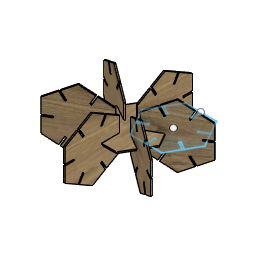
EFDI - MT03 - NDQ (Autodesk Fusion 360 design; units mm, degrees)
Autodesk Fusion 360 part; units mm, degrees
sketch "Boceto1" plane through (0, 0, 0) normal (0, 0, 1) x (1, 0, 0)
  line L0 (50, 110) -> (50, -10)
  line L1 (48.4, -10) -> (48.4, 10)
  line L2 (48.4, 10) -> (51.6, 10)
  line L3 (51.6, 10) -> (51.6, -10)
  line L4 (85.441, 31.3856) -> (102.7615, 21.3856)
  line L5 (101.1615, 18.6144) -> (83.841, 28.6144)
  line L6 (83.841, 28.6144) -> (85.441, 31.3856)
  line L7 (83.841, 71.3856) -> (101.1615, 81.3856)
  line L8 (102.7615, 78.6144) -> (85.441, 68.6144)
  line L9 (85.441, 68.6144) -> (83.841, 71.3856)
  line L10 (48.4, 90) -> (48.4, 110)
  line L11 (51.6, 110) -> (51.6, 90)
  line L12 (51.6, 90) -> (48.4, 90)
  line L13 (14.559, 68.6144) -> (-2.7615, 78.6144)
  line L14 (-1.1615, 81.3856) -> (16.159, 71.3856)
  line L15 (16.159, 71.3856) -> (14.559, 68.6144)
  line L16 (16.159, 28.6144) -> (-1.1615, 18.6144)
  line L17 (-2.7615, 21.3856) -> (14.559, 31.3856)
  line L18 (14.559, 31.3856) -> (16.159, 28.6144)
  line L19 (84.641, -10) -> (101.1615, 18.6144)
  line L20 (102.7615, 21.3856) -> (119.282, 50)
  line L21 (-19.282, 50) -> (-2.7615, 21.3856)
  line L22 (-1.1615, 18.6144) -> (15.359, -10)
  line L23 (15.359, -10) -> (48.4, -10)
  line L24 (51.6, -10) -> (84.641, -10)
  line L25 (15.359, 110) -> (-1.1615, 81.3856)
  line L26 (-2.7615, 78.6144) -> (-19.282, 50)
  line L27 (84.641, 110) -> (51.6, 110)
  line L28 (48.4, 110) -> (15.359, 110)
  line L29 (119.282, 50) -> (102.7615, 78.6144)
  line L30 (101.1615, 81.3856) -> (84.641, 110)
  point P0 (50, 50)
  point P1 (50, 50)
  point P2 (50, 50)
  point P3 (50, 50)
  point P4 (50, 50)
  point P5 (50, 50)
  dimension "d3" = 20
  dimension "d4" = 3.2
  dimension "d6" = 360
  constraint perpendicular L1 L23
  constraint perpendicular L1 L2
  constraint coincident L3.end L23
  constraint perpendicular L2 L3
  constraint symmetric L0 L1 L3
  constraint horizontal L27
  constraint collinear L19 L20
  constraint collinear L21 L22
  constraint collinear L23 L24
  constraint coincident L0.end L23
  constraint collinear L25 L26
  constraint collinear L27 L28
  constraint collinear L29 L30
  measures "d3" distance of L2 L23
  measures "d4" distance of L1 L3
extrude "Extruir1" add sketch "Boceto1" along normal mid plane 3 makes body 1
move_body "Desplazar1" bodies 1 to x (1, 0, 0) y (0, 1, 0) z (0, 0, 1) at (20, 10, 0)
copy_body "CopiarPegarCuerpos1" bodies 1 makes body 2
move_body "Desplazar2" bodies 2 to x (0, 0, 1) y (0, 1, 0) z (-1, 0, 0) at (69.5, 0, -68.5)
move_body "Desplazar4" bodies 2 to x (1, 0, 0) y (0, 1, 0) z (0, 0, 1) at (0.5, -80, -1.5)
move_body "Desplazar5" bodies 2 1 to x (1, 0, 0) y (0, 1, 0) z (0, 0, 1) at (-70, -60, 0)
pattern_circular "Patrón C1" count 6 over 360 about axis through (0, 0, 1.75) along (0, 0, 1) of bodies 2 makes body 3 at (73.9055, -44.4014, -10.747) makes body 4 at (80.779, 44.9057, 0) makes body 5 at (1.5, 93.3333, -0.5333) makes body 6 at (-74.7055, 44.8633, -11.2803) makes body 7 at (-75.4055, -41.8034, -10.747)
equation "espesor_mdf = 3 mm" comment "Espesor base para tablero de mdf a cortar."
equation "holgura_pieza = 0.1 mm" comment "Holgura para tolerancia relativa a tipo de maquina."
equation "d4 = espesor_mdf + holgura_pieza * 2"
equation "d7 = espesor_mdf"
